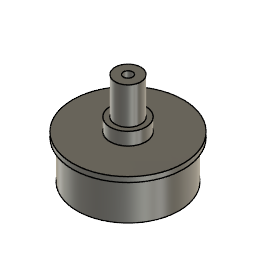
Front Wheel (Autodesk Fusion 360 design; units mm, degrees)
part number: 2026-02-27-15-49-13-223
Autodesk Fusion 360 part; units mm, degrees
sketch "Skizze1" plane through (0, 0, 0) normal (0, 0, 1) x (1, 0, 0)
  circle A0 centre (0, 0) radius 10
  circle A1 centre (0, 0) radius 9.25
  circle A2 centre (0, 0) radius 3.95
  circle A3 centre (0, 0) radius 10.85
  dimension "d1" = 20
  dimension "d2" = -0.75
  dimension "d3" = 7.9
  dimension "d4" = 1.6
  constraint coincident A0.centre A1.centre
  constraint concentric A0 A2
  measures "d1" diameter of A0
  measures "d3" diameter of A2
extrude "Extrusion1" add sketch "Skizze1" along normal blind 8.5 contours A0 | A1 | A2
sketch "Skizze4" plane through (0, 0, 8.5) normal (0, 0, 1) x (-1, 0, 0)
  circle A0 centre (0, 0) radius 10
  circle A1 centre (0, 0) radius 2.525
  circle A2 centre (0, 0) radius 3.5
  dimension "d20" = 5.05
  dimension "d21" = 7
  constraint coincident A0.centre A1.centre
  constraint concentric A1 A2
  measures "d20" diameter of A1
  measures "d21" diameter of A2
extrude "Extrusion5" add sketch "Skizze1" along normal blind 8.5 contours A3
extrude "Extrusion6" cut sketch "Skizze1" along normal blind 7.5 contours A3
extrude "Extrusion8" add sketch "Skizze4" along normal blind 9.7 contours A1
extrude "Extrusion9" add sketch "Skizze4" along normal blind 2.5 contours A2
sketch "Skizze5" plane through (0, 0, 18.2) normal (0, 0, 1) x (-1, 0, 0)
  circle A0 centre (0, 0) radius 2.525
  circle A1 centre (0, 0) radius 0.9
  dimension "d27" = 1.8
  constraint coincident A0.centre A1.centre
  measures "d27" diameter of A1
extrude "Extrusion10" cut sketch "Skizze5" against normal blind 21 contours A1
equation "d5 = 11 mm - 2.5 mm"
equation "d14 = 11 mm - 2.5 mm"
equation "d16 = 10 mm - 2.5 mm"
named bodies: "Vorderrad"
